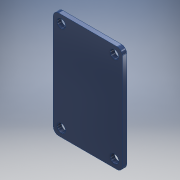
# Autodesk Inventor part: XBee mount
Saved by Autodesk Inventor 2017 (Build 210142000, 142)
## iProperties
Created: 2017-05-18
Part Number: XBee mount
Material: Generic
Document SubType Name: Modeling
Designer: yella
Density: 1 g/cm^3
Appearance: Flaked Satin - Blue
Author: yella
Autodesk Inventor part; units mm, degrees
ref_plane "YZ Plane" through (0, 0, 0) normal (1, 0, 0) x (0, 1, 0)
ref_plane "XZ Plane" through (0, 0, 0) normal (0, 1, 0) x (-1, 0, 0)
ref_plane "XY Plane" through (0, 0, 0) normal (0, 0, 1) x (1, 0, 0)
sketch "Sketch1" plane through (0, 0, 0) normal (0, 1, 0) x (-1, 0, 0)
  line L0 (-13, 18) -> (-13, -18)
  line L1 (-11, -20) -> (11, -20)
  line L2 (13, -18) -> (13, 18)
  line L3 (11, 20) -> (-11, 20)
  arc A0 (13, 18) -> (11, 20) centre (11, 18) ccw
  arc A1 (11, -20) -> (13, -18) centre (11, -18) ccw
  arc A2 (-13, -18) -> (-11, -20) centre (-11, -18) ccw
  arc A3 (-11, 20) -> (-13, 18) centre (-11, 18) ccw
  circle A4 centre (10, 17) radius 1.6
  circle A5 centre (-10, 17) radius 1.6
  circle A6 centre (10, -17) radius 1.6
  circle A7 centre (-10, -17) radius 1.6
  point P0 (13, 17)
  point P1 (-13, 17)
  point P2 (10, -20)
  point P3 (-10, -20)
  dimension "d8" = 3.2
  dimension "d11" = 3.2
  dimension "d16" = 3.2
  dimension "d17" = 3.2
  constraints: 8 centre point, 8 end point, 8 point on circle, 8 tangent, 4 point on line, 3 equal radius, 2 parallel, 1 perpendicular, 1 vertical
  measures "d8" diameter of A4
  measures "d11" diameter of A5
  measures "d16" diameter of A6
  measures "d17" diameter of A7
extrude "Extrusion1" add sketch "Sketch1" along normal blind 1.6
body "Solid1"
